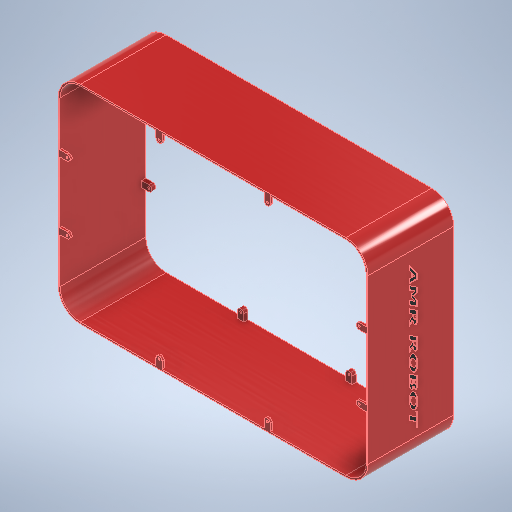
# Autodesk Inventor part: product
Saved by Autodesk Inventor 2025 (Build 290162000, 162)
## iProperties
Created: 2025-10-14
Part Number: product
Material: Generic
Document SubType Name: Modeling
Designer: hp
Density: 1 g/cm^3
Appearance: Red
Author: hp
Autodesk Inventor part; units mm, degrees
note: some values were not read from the file. Chosen so that the rebuilt part matches the saved one: direction of "Emboss1".
ref_plane "YZ Plane" through (0, 0, 0) normal (1, 0, 0) x (0, 1, 0)
ref_plane "XZ Plane" through (0, 0, 0) normal (0, 1, 0) x (-1, 0, 0)
ref_plane "XY Plane" through (0, 0, 0) normal (0, 0, 1) x (1, 0, 0)
sketch "Sketch1" plane through (0, 0, 0) normal (0, 0, 1) x (1, 0, 0)
  line L0 (-325, 250) -> (325, 250)
  line L1 (375, 200) -> (375, -200)
  line L2 (325, -250) -> (-325, -250)
  line L3 (-375, -200) -> (-375, 200)
  line L4 (-375, 250) -> (375, -250) construction
  line L5 (375, 250) -> (-375, -250) construction
  arc A0 (-325, 250) -> (-375, 200) centre (-325, 200) ccw
  arc A1 (-375, -200) -> (-325, -250) centre (-325, -200) ccw
  arc A2 (375, 200) -> (325, 250) centre (325, 200) ccw
  arc A3 (325, -250) -> (375, -200) centre (325, -200) ccw
  line L6 (325, 254) -> (-325, 254)
  arc A4 (-325, 254) -> (-379, 200) centre (-325, 200) ccw
  line L7 (-379, 200) -> (-379, -200)
  arc A5 (-379, -200) -> (-325, -254) centre (-325, -200) ccw
  line L8 (-325, -254) -> (325, -254)
  arc A6 (325, -254) -> (379, -200) centre (325, -200) ccw
  line L9 (379, -200) -> (379, 200)
  arc A7 (379, 200) -> (325, 254) centre (325, 200) ccw
  line L10 (-379, 200) -> (-375, 200)
  line L11 (-375, -200) -> (-379, -200)
  line L12 (379, 200) -> (375, 200)
  line L13 (379, -200) -> (375, -200)
  point P0 (0, 0)
  dimension "d66" = 5
  dimension "d0" = 750
  dimension "d2" = 50
  dimension "d3" = 50
  dimension "d4" = 4
  dimension "d75" = 500
  constraints: 28 end point, 16 point on circle, 9 point on line, 8 centre point, 8 tangent, 6 parallel, 3 perpendicular, 2 equal radius, 2 midpoint, 1 horizontal, 7 other
  measures "d0" distance of L4.end L5.end
  measures "d2" radius of A0
  measures "d3" radius of A3
  measures "d4" distance between parallel lines of L0 L6
  measures "d75" distance between parallel lines of L0 L2
extrude "Extrusion1" add sketch "Sketch1" along normal blind 210 contours A0 L10 A4 L6 A7 L12 A2 L0 | L3 L11 L7 L10 | L12 L9 L13 L1 | A1 L2 A3 L13 A6 L8 A5 L11
sketch "Sketch2" plane through (0, 0, 210) normal (0, 0, 1) x (1, 0, 0)
  line L0 (-325, 250) -> (325, 250) projected
  line L1 (-140, 250) -> (-125, 250)
  line L2 (-125, -250) -> (-140, -250)
  line L3 (125, 250) -> (140, 250)
  line L4 (140, -250) -> (125, -250)
  line L5 (-375, -200) -> (-375, 200) projected
  line L6 (375, 90) -> (375, 75)
  line L7 (-375, 75) -> (-375, 90)
  line L8 (375, 200) -> (375, -200) projected
  line L9 (375, -75) -> (375, -90)
  line L10 (325, -250) -> (-325, -250) projected
  line L11 (125, 232.5) -> (125, 250)
  line L12 (140, 250) -> (140, 232.5)
  line L13 (-125, 250) -> (-125, 232.5)
  line L14 (-140, 232.5) -> (-140, 250)
  line L15 (-375, 90) -> (-357.5, 90)
  line L16 (-357.5, 75) -> (-375, 75)
  line L17 (-375, -75) -> (-357.5, -75)
  line L18 (-357.5, -90) -> (-375, -90)
  line L19 (-140, -250) -> (-140, -232.5)
  line L20 (-125, -232.5) -> (-125, -250)
  line L21 (140, -232.5) -> (140, -250)
  line L22 (125, -250) -> (125, -232.5)
  line L23 (357.5, -75) -> (375, -75)
  line L24 (375, -90) -> (357.5, -90)
  line L25 (357.5, 90) -> (375, 90)
  line L26 (375, 75) -> (357.5, 75)
  arc A0 (-140, 232.5) -> (-125, 232.5) centre (-132.5, 232.5) ccw
  arc A1 (125, 232.5) -> (140, 232.5) centre (132.5, 232.5) ccw
  arc A2 (-357.5, 75) -> (-357.5, 90) centre (-357.5, 82.5) ccw
  arc A3 (-357.5, -90) -> (-357.5, -75) centre (-357.5, -82.5) ccw
  arc A4 (-125, -232.5) -> (-140, -232.5) centre (-132.5, -232.5) ccw
  arc A5 (140, -232.5) -> (125, -232.5) centre (132.5, -232.5) ccw
  arc A6 (357.5, -75) -> (357.5, -90) centre (357.5, -82.5) ccw
  arc A7 (357.5, 90) -> (357.5, 75) centre (357.5, 82.5) ccw
  circle A8 centre (132.5, 232.5) radius 2.5
  circle A9 centre (-132.5, 232.5) radius 2.5
  circle A10 centre (-357.5, 82.5) radius 2.5
  circle A11 centre (-357.5, -82.5) radius 2.5
  circle A12 centre (-132.5, -232.5) radius 2.5
  circle A13 centre (132.5, -232.5) radius 2.5
  circle A14 centre (357.5, -82.5) radius 2.5
  circle A15 centre (357.5, 82.5) radius 2.5
  point P0 (-132.5, -250)
  point P1 (132.5, -250)
  point P2 (-362.5, 75)
  point P3 (362.5, -75)
  point P4 (362.5, 75)
  point P5 (362.5, -90)
  point P6 (125, -187.5)
  point P7 (-140, -187.5)
  point P8 (375, -75)
  point P9 (-375, -90)
  point P10 (140, 250)
  point P11 (-125, 250)
  point P12 (-375, 82.5)
  point P13 (-132.5, -225)
  point P14 (375, -82.5)
  dimension "d32" = 750
  dimension "d33" = 15
  dimension "d48" = 0
  dimension "d50" = 250
  dimension "d51" = 235
  dimension "d53" = 15
  dimension "d54" = 15
  dimension "d55" = 150
  dimension "d56" = 160
  dimension "d57" = 15
  dimension "d58" = 150
  dimension "d59" = 160
  dimension "d60" = 15
  dimension "d61" = 15
  dimension "d62" = 250
  dimension "d63" = 250
  dimension "d64" = 15
  dimension "d65" = 5
  dimension "d66" = 5
  dimension "d67" = 5
  dimension "d68" = 5
  dimension "d69" = 5
  dimension "d70" = 5
  dimension "d71" = 5
  dimension "d72" = 5
  dimension "d76" = 17.5
  dimension "d78" = 17.5
  dimension "d79" = 17.5
  dimension "d80" = 15
  dimension "d81" = 17.5
  dimension "d82" = 17.5
  dimension "d83" = 25
  dimension "d84" = 17.5
  dimension "d85" = 17.5
  constraints: 46 end point, 19 parallel, 17 point on circle, 16 centre point, 16 tangent, 12 point on line, 8 coincident, 8 perpendicular, 6 horizontal, 4 midpoint, 1 collinear
  measures "d32" distance of L7.end L6.start
  measures "d33" distance of L6.start L6.end
  measures "d48" distance from line of L10 point (-132.5, -250)
  measures "d50" distance from line of L3.start L13
  measures "d51" distance between parallel lines of L8 L12
  measures "d53" distance from line of L3.end L11
  measures "d54" distance between parallel lines of L16 L15
  measures "d55" distance from line of L17 point (-362.5, 75)
  measures "d56" distance between parallel lines of L10 L18
  measures "d57" distance between parallel lines of L18 L17
  measures "d58" distance of point (362.5, -75) point (362.5, 75)
  measures "d59" distance from line of L10 point (362.5, -90)
  measures "d60" distance between parallel lines of L24 L23
  measures "d61" distance from line of point (125, -187.5) L21
  measures "d62" distance from line of L8 point (125, -187.5)
  measures "d63" distance between parallel lines of L22 L20
  measures "d64" distance from line of L20 point (-140, -187.5)
  measures "d65" diameter of A8
  measures "d66" diameter of A9
  measures "d67" diameter of A10
  measures "d68" diameter of A11
  measures "d69" diameter of A12
  measures "d70" diameter of A13
  measures "d71" diameter of A14
  measures "d72" diameter of A15
  measures "d76" distance from line of L4 A5.centre
  measures "d78" distance from line of A1.centre L3
  measures "d79" distance from line of A0.centre L0
  measures "d80" distance between parallel lines of L13 L14
  measures "d81" distance of point (-375, 82.5) A2.centre
  measures "d82" distance from line of L5 A3.centre
  measures "d83" distance from line of L10 point (-132.5, -225)
  measures "d84" distance of point (375, -82.5) A6.centre
  measures "d85" distance from line of A7.centre L6
extrude "Extrusion2" add sketch "Sketch2" against normal blind 5
sketch "Sketch3" plane through (379, -200, 0) normal (1, 0, 0) x (0, 0, -1)
  line L0 (-207.776, 400) -> (-207.776, -1.3337)
  line L1 (-207.776, -1.3337) -> (0, -1.3337)
  line L2 (0, -1.3337) -> (0, 400)
  line L3 (0, 400) -> (-207.776, 400)
  line L4 (0, 0) -> (0, 400) projected
  line L5 (-108.3173, 370.3786) -> (-88.3173, 343.2473)
  line L6 (-88.3173, 343.2473) -> (-88.3173, 332.291)
  line L7 (-88.3173, 332.291) -> (-108.3173, 332.3721)
  line L8 (-108.3173, 332.3721) -> (-108.3173, 342.7124)
  line L9 (-108.3173, 342.7124) -> (-104.2331, 342.4369)
  line L10 (-104.2331, 342.4369) -> (-104.2331, 355.0301)
  line L11 (-104.2331, 355.0301) -> (-108.3173, 360.2975)
  line L12 (-108.3173, 360.2975) -> (-108.3173, 370.3786)
  line L13 (-100.6026, 342.1776) -> (-94.0062, 341.7724)
  line L14 (-94.0062, 341.7724) -> (-100.6026, 350.3461)
  line L15 (-100.6026, 350.3461) -> (-100.6026, 342.1776)
  line L16 (-108.3173, 287.4936) -> (-108.3173, 297.4936)
  line L17 (-108.3173, 297.4936) -> (-95.0596, 288.4823)
  line L18 (-95.0596, 288.4823) -> (-103.6172, 301.5941)
  line L19 (-103.6172, 301.5941) -> (-103.6172, 308.4499)
  line L20 (-103.6172, 308.4499) -> (-95.0596, 309.9247)
  line L21 (-95.0596, 309.9247) -> (-108.3173, 318.9361)
  line L22 (-108.3173, 318.9361) -> (-108.3173, 328.4012)
  line L23 (-108.3173, 328.4012) -> (-88.3173, 314.8032)
  line L24 (-88.3173, 314.8032) -> (-88.3173, 303.1987)
  line L25 (-88.3173, 303.1987) -> (-98.1877, 301.0431)
  line L26 (-98.1877, 301.0431) -> (-88.3173, 285.4839)
  line L27 (-88.3173, 285.4839) -> (-88.3173, 273.8956)
  line L28 (-88.3173, 273.8956) -> (-108.3173, 287.4936)
  line L29 (-108.3173, 242.21) -> (-108.3173, 254.4628)
  line L30 (-108.3173, 254.4628) -> (-100.9754, 260.6379)
  line L31 (-100.9754, 260.6379) -> (-100.9754, 264.2359)
  line L32 (-100.9754, 264.2359) -> (-108.3173, 269.2278)
  line L33 (-108.3173, 269.2278) -> (-108.3173, 279.2278)
  line L34 (-108.3173, 279.2278) -> (-88.3173, 265.6298)
  line L35 (-88.3173, 265.6298) -> (-88.3173, 249.5196)
  spline S0 degree 2 poles (-88.3173, 249.5196) (-88.3173, 246.197) (-88.7387, 241.5293) (-89.387, 239.8761) knots 0 0 0 1 2 2 2
  spline S1 degree 2 poles (-89.387, 239.8761) (-90.0678, 238.1905) (-92.1909, 237.1046) (-93.8117, 238.2068) knots 0 0 0 1 2 2 2
  spline S2 degree 2 poles (-93.8117, 238.2068) (-96.0969, 239.7627) (-98.9656, 245.8567) (-99.8084, 249.8923) knots 0 0 0 1 2 2 2
  line L36 (-99.8084, 249.8923) -> (-108.3173, 242.21)
  spline S3 degree 2 poles (-94.4438, 248.9523) (-93.682, 248.4499) (-92.5961, 248.8713) (-92.3044, 250.0058) knots 0 0 0 1 2 2 2
  spline S4 degree 2 poles (-92.3044, 250.0058) (-92.1099, 250.8162) (-91.9964, 253.0528) (-91.9964, 254.7708) knots 0 0 0 1 2 2 2
  line L37 (-91.9964, 254.7708) -> (-91.9964, 258.1257)
  line L38 (-91.9964, 258.1257) -> (-97.3773, 261.7886)
  line L39 (-97.3773, 261.7886) -> (-97.3773, 258.9037)
  spline S5 degree 2 poles (-97.3773, 258.9037) (-97.3773, 256.8129) (-97.118, 253.7173) (-96.7128, 252.4045) knots 0 0 0 1 2 2 2
  spline S6 degree 2 poles (-96.7128, 252.4045) (-96.3238, 251.1889) (-95.2866, 249.5358) (-94.4438, 248.9523) knots 0 0 0 1 2 2 2
  line L40 (-108.3173, 186.116) -> (-108.3173, 198.3688)
  line L41 (-108.3173, 198.3688) -> (-100.9754, 204.5439)
  line L42 (-100.9754, 204.5439) -> (-100.9754, 208.1419)
  line L43 (-100.9754, 208.1419) -> (-108.3173, 213.1338)
  line L44 (-108.3173, 213.1338) -> (-108.3173, 223.1338)
  line L45 (-108.3173, 223.1338) -> (-88.3173, 209.5358)
  line L46 (-88.3173, 209.5358) -> (-88.3173, 193.4256)
  spline S7 degree 2 poles (-88.3173, 193.4256) (-88.3173, 190.103) (-88.7387, 185.4353) (-89.387, 183.7821) knots 0 0 0 1 2 2 2
  spline S8 degree 2 poles (-89.387, 183.7821) (-90.0678, 182.0965) (-92.1909, 181.0106) (-93.8117, 182.1128) knots 0 0 0 1 2 2 2
  spline S9 degree 2 poles (-93.8117, 182.1128) (-96.0969, 183.6687) (-98.9656, 189.7627) (-99.8084, 193.7983) knots 0 0 0 1 2 2 2
  line L47 (-99.8084, 193.7983) -> (-108.3173, 186.116)
  spline S10 degree 2 poles (-94.4438, 192.8583) (-93.682, 192.3559) (-92.5961, 192.7773) (-92.3044, 193.9118) knots 0 0 0 1 2 2 2
  spline S11 degree 2 poles (-92.3044, 193.9118) (-92.1099, 194.7222) (-91.9964, 196.9588) (-91.9964, 198.6768) knots 0 0 0 1 2 2 2
  line L48 (-91.9964, 198.6768) -> (-91.9964, 202.0317)
  line L49 (-91.9964, 202.0317) -> (-97.3773, 205.6946)
  line L50 (-97.3773, 205.6946) -> (-97.3773, 202.8097)
  spline S12 degree 2 poles (-97.3773, 202.8097) (-97.3773, 200.7189) (-97.118, 197.6233) (-96.7128, 196.3105) knots 0 0 0 1 2 2 2
  spline S13 degree 2 poles (-96.7128, 196.3105) (-96.3238, 195.0949) (-95.2866, 193.4418) (-94.4438, 192.8583) knots 0 0 0 1 2 2 2
  spline S14 degree 2 poles (-98.3173, 139.9085) (-103.1796, 143.1987) (-108.7387, 157.364) (-108.7387, 166.4077) knots 0 0 0 1 2 2 2
  spline S15 degree 2 poles (-108.7387, 166.4077) (-108.7387, 175.4677) (-103.1148, 181.9507) (-98.3173, 178.7092) knots 0 0 0 1 2 2 2
  spline S16 degree 2 poles (-98.3173, 178.7092) (-93.5037, 175.4191) (-87.896, 161.2862) (-87.896, 152.2262) knots 0 0 0 1 2 2 2
  spline S17 degree 2 poles (-87.896, 152.2262) (-87.896, 143.1824) (-93.4713, 136.6022) (-98.3173, 139.9085) knots 0 0 0 1 2 2 2
  spline S18 degree 2 poles (-98.3173, 150.2651) (-96.5183, 149.0495) (-94.0062, 148.8226) (-93.212, 149.5034) knots 0 0 0 1 2 2 2
  spline S19 degree 2 poles (-93.212, 149.5034) (-92.3854, 150.2489) (-91.6723, 153.0204) (-91.6723, 154.7708) knots 0 0 0 1 2 2 2
  spline S20 degree 2 poles (-91.6723, 154.7708) (-91.6723, 156.6184) (-92.3368, 160.0868) (-93.1796, 162.0641) knots 0 0 0 1 2 2 2
  spline S21 degree 2 poles (-93.1796, 162.0641) (-93.9575, 163.8307) (-96.5345, 167.1209) (-98.3173, 168.3364) knots 0 0 0 1 2 2 2
  spline S22 degree 2 poles (-98.3173, 168.3364) (-100.165, 169.5844) (-102.5961, 169.7789) (-103.4227, 169.082) knots 0 0 0 1 2 2 2
  spline S23 degree 2 poles (-103.4227, 169.082) (-104.2493, 168.3526) (-104.9624, 165.5487) (-104.9624, 163.7983) knots 0 0 0 1 2 2 2
  spline S24 degree 2 poles (-104.9624, 163.7983) (-104.9624, 162.0317) (-104.2007, 158.1743) (-103.3903, 156.4077) knots 0 0 0 1 2 2 2
  spline S25 degree 2 poles (-103.3903, 156.4077) (-102.5151, 154.5277) (-100.1974, 151.5455) (-98.3173, 150.2651) knots 0 0 0 1 2 2 2
  spline S26 degree 2 poles (-102.1909, 104.5925) (-103.682, 105.5974) (-105.9348, 109.3899) (-106.6804, 111.8048) knots 0 0 0 1 2 2 2
  spline S27 degree 2 poles (-106.6804, 111.8048) (-107.5718, 114.6735) (-108.3173, 120.5893) (-108.3173, 124.7546) knots 0 0 0 1 2 2 2
  line L51 (-108.3173, 124.7546) -> (-108.3173, 140.7675)
  line L52 (-108.3173, 140.7675) -> (-88.3173, 127.1695)
  line L53 (-88.3173, 127.1695) -> (-88.3173, 113.0204)
  spline S28 degree 2 poles (-88.3173, 113.0204) (-88.3173, 108.6119) (-88.6577, 104.3008) (-89.1925, 102.68) knots 0 0 0 1 2 2 2
  spline S29 degree 2 poles (-89.1925, 102.68) (-89.7598, 100.9134) (-91.7047, 100.1192) (-92.9689, 100.962) knots 0 0 0 1 2 2 2
  spline S30 degree 2 poles (-92.9689, 100.962) (-94.4276, 101.9669) (-96.7128, 106.4401) (-97.2477, 109.3899) knots 0 0 0 1 2 2 2
  line L54 (-97.2477, 109.3899) -> (-97.3449, 109.4709)
  spline S31 degree 2 poles (-97.3449, 109.4709) (-97.7339, 106.0187) (-100.1488, 103.1987) (-102.1909, 104.5925) knots 0 0 0 1 2 2 2
  spline S32 degree 2 poles (-102.1099, 114.8842) (-101.1699, 114.2521) (-100.1164, 115.0463) (-99.8408, 116.3591) knots 0 0 0 1 2 2 2
  spline S33 degree 2 poles (-99.8408, 116.3591) (-99.6626, 117.1533) (-99.6301, 120.3137) (-99.6301, 123.0042) knots 0 0 0 1 2 2 2
  line L55 (-99.6301, 123.0042) -> (-99.6301, 124.8518)
  line L56 (-99.6301, 124.8518) -> (-104.6707, 128.2878)
  line L57 (-104.6707, 128.2878) -> (-104.6707, 127.7529)
  spline S34 degree 2 poles (-104.6707, 127.7529) (-104.6707, 123.8307) (-104.622, 120.7837) (-104.2817, 119.0009) knots 0 0 0 1 2 2 2
  spline S35 degree 2 poles (-104.2817, 119.0009) (-103.9737, 117.4288) (-102.8392, 115.3867) (-102.1099, 114.8842) knots 0 0 0 1 2 2 2
  spline S36 degree 2 poles (-93.9575, 111.8534) (-93.4713, 111.5293) (-92.4502, 111.821) (-92.2233, 112.7124) knots 0 0 0 1 2 2 2
  spline S37 degree 2 poles (-92.2233, 112.7124) (-91.9964, 113.5714) (-91.964, 116.2619) (-91.964, 118.9523) knots 0 0 0 1 2 2 2
  line L58 (-91.964, 118.9523) -> (-91.964, 119.6492)
  line L59 (-91.964, 119.6492) -> (-96.2104, 122.5341)
  line L60 (-96.2104, 122.5341) -> (-96.2104, 121.27)
  spline S38 degree 2 poles (-96.2104, 121.27) (-96.2104, 118.693) (-96.1618, 116.586) (-95.9024, 115.3056) knots 0 0 0 1 2 2 2
  spline S39 degree 2 poles (-95.9024, 115.3056) (-95.6107, 113.8956) (-94.622, 112.3072) (-93.9575, 111.8534) knots 0 0 0 1 2 2 2
  spline S40 degree 2 poles (-98.3173, 59.7465) (-103.1796, 63.0366) (-108.7387, 77.2019) (-108.7387, 86.2457) knots 0 0 0 1 2 2 2
  spline S41 degree 2 poles (-108.7387, 86.2457) (-108.7387, 95.3056) (-103.1148, 101.7886) (-98.3173, 98.5471) knots 0 0 0 1 2 2 2
  spline S42 degree 2 poles (-98.3173, 98.5471) (-93.5037, 95.257) (-87.896, 81.1241) (-87.896, 72.0641) knots 0 0 0 1 2 2 2
  spline S43 degree 2 poles (-87.896, 72.0641) (-87.896, 63.0204) (-93.4713, 56.4401) (-98.3173, 59.7465) knots 0 0 0 1 2 2 2
  spline S44 degree 2 poles (-98.3173, 70.103) (-96.5183, 68.8875) (-94.0062, 68.6606) (-93.212, 69.3413) knots 0 0 0 1 2 2 2
  spline S45 degree 2 poles (-93.212, 69.3413) (-92.3854, 70.0868) (-91.6723, 72.8583) (-91.6723, 74.6087) knots 0 0 0 1 2 2 2
  spline S46 degree 2 poles (-91.6723, 74.6087) (-91.6723, 76.4564) (-92.3368, 79.9247) (-93.1796, 81.9021) knots 0 0 0 1 2 2 2
  spline S47 degree 2 poles (-93.1796, 81.9021) (-93.9575, 83.6687) (-96.5345, 86.9588) (-98.3173, 88.1743) knots 0 0 0 1 2 2 2
  spline S48 degree 2 poles (-98.3173, 88.1743) (-100.165, 89.4223) (-102.5961, 89.6168) (-103.4227, 88.9199) knots 0 0 0 1 2 2 2
  spline S49 degree 2 poles (-103.4227, 88.9199) (-104.2493, 88.1905) (-104.9624, 85.3867) (-104.9624, 83.6363) knots 0 0 0 1 2 2 2
  spline S50 degree 2 poles (-104.9624, 83.6363) (-104.9624, 81.8696) (-104.2007, 78.0123) (-103.3903, 76.2457) knots 0 0 0 1 2 2 2
  spline S51 degree 2 poles (-103.3903, 76.2457) (-102.5151, 74.3656) (-100.1974, 71.3834) (-98.3173, 70.103) knots 0 0 0 1 2 2 2
  line L61 (-108.3173, 52.9069) -> (-92.1261, 41.8858)
  line L62 (-92.1261, 41.8858) -> (-92.1261, 53.7173)
  line L63 (-92.1261, 53.7173) -> (-88.3173, 51.1403)
  line L64 (-88.3173, 51.1403) -> (-88.3173, 17.4288)
  line L65 (-88.3173, 17.4288) -> (-92.1261, 20.0058)
  line L66 (-92.1261, 20.0058) -> (-92.1261, 31.8372)
  line L67 (-92.1261, 31.8372) -> (-108.3173, 42.8583)
  line L68 (-108.3173, 42.8583) -> (-108.3173, 52.9069)
  point P0 (0, 200)
  constraints: 1 coincident, 1 collinear, 2 other
sketch "Sketch4" plane through (0, 0, 0) normal (0, 0, -1) x (-1, 0, 0)
  line L0 (-325, 250) -> (325, 250)
  line L1 (-140, 250) -> (-125, 250)
  line L2 (-125, -250) -> (-140, -250)
  line L3 (125, 250) -> (140, 250)
  line L4 (140, -250) -> (125, -250)
  line L5 (-375, -209.7168) -> (-375, 129.8759)
  line L6 (375, 90) -> (375, 75)
  line L7 (-375, 75) -> (-375, 90)
  line L8 (375, 166.9694) -> (375, -233.0306)
  line L9 (375, -75) -> (375, -90)
  line L10 (254.1053, -250) -> (-395.8947, -250)
  line L11 (125, 232.5) -> (125, 250)
  line L12 (140, 250) -> (140, 232.5)
  line L13 (-125, 250) -> (-125, 232.5)
  line L14 (-140, 232.5) -> (-140, 250)
  line L15 (-375, 90) -> (-357.5, 90)
  line L16 (-357.5, 75) -> (-375, 75)
  line L17 (-375, -75) -> (-357.5, -75)
  line L18 (-357.5, -90) -> (-445.8947, -90)
  line L19 (-140, -250) -> (-140, -232.5)
  line L20 (-125, -232.5) -> (-125, -250)
  line L21 (140, -232.5) -> (140, -250)
  line L22 (125, -250) -> (125, -232.5)
  line L23 (357.5, -75) -> (375, -75)
  line L24 (375, -90) -> (357.5, -90)
  line L25 (357.5, 90) -> (375, 90)
  line L26 (375, 75) -> (357.5, 75)
  arc A0 (-140, 232.5) -> (-125, 232.5) centre (-132.5, 232.5) ccw
  arc A1 (125, 232.5) -> (140, 232.5) centre (132.5, 232.5) ccw
  arc A2 (-357.5, 75) -> (-357.5, 90) centre (-357.5, 82.5) ccw
  arc A3 (-357.5, -90) -> (-357.5, -75) centre (-357.5, -82.5) ccw
  arc A4 (-125, -232.5) -> (-140, -232.5) centre (-132.5, -232.5) ccw
  arc A5 (140, -232.5) -> (125, -232.5) centre (132.5, -232.5) ccw
  arc A6 (357.5, -75) -> (357.5, -90) centre (357.5, -82.5) ccw
  arc A7 (357.5, 90) -> (357.5, 75) centre (357.5, 82.5) ccw
  circle A8 centre (132.5, 232.5) radius 2.5
  circle A9 centre (-132.5, 232.5) radius 2.5
  circle A10 centre (-357.5, 82.5) radius 2.5
  circle A11 centre (-357.5, -82.5) radius 2.5
  circle A12 centre (-132.5, -232.5) radius 2.5
  circle A13 centre (132.5, -232.5) radius 2.5
  circle A14 centre (357.5, -82.5) radius 2.5
  circle A15 centre (357.5, 82.5) radius 2.5
  line L27 (375, -200) -> (375, 200) projected
  line L28 (-325, -250) -> (325, -250) projected
  line L29 (325, 250) -> (-325, 250) projected
  line L30 (-375, 200) -> (-375, -200) projected
  point P0 (0, 0)
  point P1 (-132.5, -250)
  point P2 (132.5, -250)
  point P3 (-433.3947, 75)
  point P4 (291.6053, -75)
  point P5 (291.6053, 75)
  point P6 (291.6053, -90)
  point P7 (125, -220.5306)
  point P8 (-140, -220.5306)
  point P9 (-375, 82.5)
  point P10 (-132.5, -225)
  point P11 (375, -82.5)
  point P12 (-375, -90)
  dimension "d86" = 750
  dimension "d87" = 15
  dimension "d88" = 0
  dimension "d89" = 250
  dimension "d90" = 235
  dimension "d91" = 15
  dimension "d92" = 15
  dimension "d93" = 150
  dimension "d94" = 160
  dimension "d95" = 15
  dimension "d96" = 150
  dimension "d97" = 160
  dimension "d98" = 15
  dimension "d99" = 15
  dimension "d100" = 250
  dimension "d101" = 250
  dimension "d102" = 15
  dimension "d103" = 5
  dimension "d104" = 5
  dimension "d105" = 5
  dimension "d106" = 5
  dimension "d107" = 5
  dimension "d108" = 5
  dimension "d109" = 5
  dimension "d110" = 5
  dimension "d111" = 17.5
  dimension "d112" = 17.5
  dimension "d113" = 17.5
  dimension "d114" = 15
  dimension "d115" = 17.5
  dimension "d116" = 17.5
  dimension "d117" = 25
  dimension "d118" = 17.5
  dimension "d119" = 17.5
  dimension "d120" = 375
  constraints: 54 end point, 19 parallel, 17 point on circle, 16 centre point, 16 tangent, 12 point on line, 8 coincident, 8 perpendicular, 6 horizontal, 5 collinear, 4 midpoint
  measures "d86" distance of L7.end L6.start
  measures "d87" distance of L6.start L6.end
  measures "d88" distance from line of L10 point (-132.5, -250)
  measures "d89" distance from line of L3.start L13
  measures "d90" distance between parallel lines of L8 L12
  measures "d91" distance from line of L3.end L11
  measures "d92" distance between parallel lines of L16 L15
  measures "d93" distance from line of L17 point (-433.395, 75)
  measures "d94" distance between parallel lines of L10 L18
  measures "d95" distance between parallel lines of L18 L17
  measures "d96" distance of point (291.605, -75) point (291.605, 75)
  measures "d97" distance from line of L10 point (291.605, -90)
  measures "d98" distance between parallel lines of L24 L23
  measures "d99" distance from line of point (125, -220.531) L21
  measures "d100" distance from line of L8 point (125, -220.531)
  measures "d101" distance between parallel lines of L22 L20
  measures "d102" distance from line of L20 point (-140, -220.531)
  measures "d103" diameter of A8
  measures "d104" diameter of A9
  measures "d105" diameter of A10
  measures "d106" diameter of A11
  measures "d107" diameter of A12
  measures "d108" diameter of A13
  measures "d109" diameter of A14
  measures "d110" diameter of A15
  measures "d111" distance from line of L4 A5.centre
  measures "d112" distance from line of A1.centre L3
  measures "d113" distance from line of A0.centre L0
  measures "d114" distance between parallel lines of L13 L14
  measures "d115" distance of point (-375, 82.5) A2.centre
  measures "d116" distance from line of L5 A3.centre
  measures "d117" distance from line of L10 point (-132.5, -225)
  measures "d118" distance of point (375, -82.5) A6.centre
  measures "d119" distance from line of A7.centre L6
  measures "d120" distance from line of point (0, 0) L8
extrude "Extrusion3" add sketch "Sketch4" against normal blind 10
emboss "Emboss1" sketch "Sketch3" operation cut depth 2 direction (-1, 0, 0) contours L5 L6 L7 L8 L9 L10 L11 L12 | L16 L17 L18 L19 L20 L21 L22 L23 L24 L25 L26 L27 L28 | L29 L30 L31 L32 L33 L34 L35 S0 S1 S2 L36 | L40 L41 L42 L43 L44 L45 L46 S7 S8 S9 L47 | S14 S15 S16 S17 | S26 S27 L51 L52 L53 S28 S29 S30 L54 S31 | S40 S41 S42 S43 | L61 L62 L63 L64 L65 L66 L67 L68
body "Solid1"
